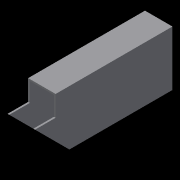
# Autodesk Inventor part: Bumper Rail Stand
Saved by Autodesk Inventor 2014 SP1 (Build 180222100, 222)
## iProperties
Created: 2013-11-29
Part Number: Bumper Rail Stand
Material: Generic
Document SubType Name: Modeling
Designer: Rauhul Varma
Mass: 24.9287 g
Surface Area: 319.842 cm^2
Volume: 24.9287 cm^3
Density: 1 g/cm^3
Appearance: Default
Author: Rauhul Varma
Autodesk Inventor part; units mm, degrees
ref_plane "YZ Plane" through (0, 0, 0) normal (1, 0, 0) x (0, 1, 0)
ref_plane "XZ Plane" through (0, 0, 0) normal (0, 1, 0) x (-1, 0, 0)
ref_plane "XY Plane" through (0, 0, 0) normal (0, 0, 1) x (1, 0, 0)
sketch "Sketch1" plane through (0, 0, 0) normal (0, 0, 1) x (1, 0, 0)
  line L0 (0, 0) -> (25.4, 0)
  line L1 (25.4, 0) -> (25.4, 50.8)
  line L2 (25.4, 50.8) -> (0, 50.8)
  line L3 (0, 50.8) -> (0, 0)
  line L4 (1.5875, 1.5875) -> (23.8125, 1.5875)
  line L5 (23.8125, 1.5875) -> (23.8125, 49.2125)
  line L6 (23.8125, 49.2125) -> (1.5875, 49.2125)
  line L7 (1.5875, 49.2125) -> (1.5875, 1.5875)
  dimension "d0" = 25.4
  dimension "d1" = 50.8
  dimension "d2" = 1.5875
  dimension "d3" = 1.5875
  dimension "d4" = 1.5875
  dimension "d5" = 1.5875
  constraints: 16 end point, 4 parallel, 2 horizontal, 2 perpendicular
  measures "d0" distance of L2.end L1.end
  measures "d1" distance of L1.end L0.end
  measures "d2" distance between parallel lines of L2 L6
  measures "d3" distance between parallel lines of L1 L5
  measures "d4" distance between parallel lines of L3 L7
  measures "d5" distance between parallel lines of L0 L4
extrude "Box Beam Profile" add sketch "Sketch1" along normal blind 127
sketch "Sketch2" plane through (25.4, 0, 0) normal (1, 0, 0) x (0, 0, -1)
  line L0 (0, 50.8) -> (-127, 50.8) projected
  line L1 (-127, 0) -> (-127, 50.8) projected
  line L2 (0, 0) -> (-127, 0) projected
  line L3 (-127, 31.75) -> (-95.25, 0)
  line L4 (-127, 31.75) -> (-107.95, 31.75)
  line L5 (-107.95, 31.75) -> (-107.95, 50.8)
  dimension "d8" = 45
  dimension "d9" = 19.05
  dimension "d10" = 19.05
  constraints: 6 end point, 3 point on line, 1 parallel, 1 perpendicular
  measures "d8" angle of L1 L3
  measures "d9" distance of L0.end L3.start
  measures "d10" distance of L3.start L4.end
extrude "Through Cutouts" cut sketch "Sketch2" against normal through all
equation "\"d3\" = d2"
equation "\"d4\" = d2"
equation "\"d5\" = d2"
equation "\"d10\" = d9"
body "Solid1"
